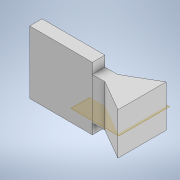
# Autodesk Inventor part: Scheibengeometrie_einfach
Saved by Autodesk Inventor 2020 (Build 240168000, 168)
## iProperties
Created: 2019-07-21
Part Number: Scheibengeometrie_einfach
Material: Generisch
Document SubType Name: Modeling
Designer: Limmer
Density: 1 g/cm^3
Appearance: Vorgabe
Author: Limmer
Autodesk Inventor part; units mm, degrees
ref_plane "YZ Plane" through (0, 0, 0) normal (1, 0, 0) x (0, 1, 0)
ref_plane "XZ Plane" through (0, 0, 0) normal (0, 1, 0) x (-1, 0, 0)
ref_plane "XY Plane" through (0, 0, 0) normal (0, 0, 1) x (1, 0, 0)
sketch "Skizze1" plane through (0, 0, 0) normal (0, 1, 0) x (-1, 0, 0)
  line L0 (0, 0) -> (0, -5.75)
  line L1 (0, 0) -> (0, 5.75)
  line L2 (0, 5.75) -> (6.7337, 5.75) construction
  line L3 (0, 5.75) -> (7.3612, 1.5)
  line L4 (0, 5.75) -> (11, 5.75) construction
  line L5 (7.3612, -1.5) -> (0, -5.75)
  line L6 (7.3612, 1.5) -> (6.8494, 1.7955)
  line L7 (7.3612, 1.5) -> (10.3612, 1.5)
  line L8 (10.3612, 1.5) -> (10.3612, -1.5)
  line L9 (10.3612, -1.5) -> (7.3612, -1.5)
  dimension "d0" = 5.75
  dimension "d1" = 5.75
  dimension "d5" = 30
  dimension "d8" = 3
  constraints: 20 end point, 3 horizontal, 2 vertical, 1 parallel, 1 perpendicular, 1 point on line
  measures "d0" distance of L0.start L0.end
  measures "d1" distance of L0.start L1.end
  measures "d5" angle of L3 L4
  measures "d8" distance of L5.start L8.end
extrude "Extrusion1" add sketch "Skizze1" along normal blind 10
ref_plane "Arbeitsebene1" through (0, 5, 0) normal (0, 1, 0) x (1, 0, 0)
sketch "Skizze2" plane through (0, 5, 0) normal (0, 1, 0) x (1, 0, 0)
  line L0 (-7.3612, 1.5) -> (-10.3612, 1.5) projected
  line L1 (-10.3612, 1.5) -> (-25.3612, 1.5)
  line L2 (-10.3612, -1.45) -> (-10.3612, 1.5)
  line L3 (-10.3612, 1.5) -> (-10.3612, -1.5) projected
  line L4 (-10.3612, -1.5) -> (-25.3612, -1.45)
  line L5 (-25.3612, 1.5) -> (-25.3612, -1.45)
  point P0 (0, 0)
  dimension "d12" = 15
  constraints: 8 end point, 1 horizontal, 1 vertical
  measures "d12" distance of L2.start L4.end
extrude "Extrusion2" add sketch "Skizze2" along normal mid plane 15
